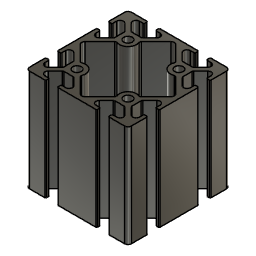
DLLPDF 153030 Cube (Autodesk Fusion 360 design; units mm, degrees)
part number: DLLPDF-153030-350-A
Autodesk Fusion 360 part; units mm, degrees
sketch "Sketch1" plane through (0, 0, 0) normal (0, 0, 1) x (1, 0, 0)
  line L0 (-2.5, 1.5491) -> (-4.7083, 3.7573)
  arc A0 (-4.7083, 3.7573) -> (-6.4, 3.0566) centre (-5.409, 3.0566) ccw
  line L1 (-6.4, 1.95) -> (-6.4, 3.0566)
  arc A1 (-6.65, 1.7) -> (-6.4, 1.95) centre (-6.65, 1.95) ccw
  line L2 (-7.25, 1.7) -> (-6.65, 1.7)
  arc A2 (-7.5, 1.95) -> (-7.25, 1.7) centre (-7.25, 1.95) ccw
  line L3 (-7.5, -6.5) -> (-7.5, -1.95)
  arc A3 (-7.5, -6.5) -> (-6.5, -7.5) centre (-6.5, -6.5) ccw
  line L4 (-6.5, -7.5) -> (-1.95, -7.5)
  arc A4 (-1.95, -7.5) -> (-1.7, -7.25) centre (-1.95, -7.25) ccw
  line L5 (-1.7, -7.25) -> (-1.7, -6.65)
  line L6 (-1.95, -6.4) -> (-3.0566, -6.4)
  arc A5 (-1.7, -6.65) -> (-1.95, -6.4) centre (-1.95, -6.65) ccw
  arc A6 (-3.7573, -4.7083) -> (-3.0566, -6.4) centre (-3.0566, -5.409) ccw
  line L7 (-1.5491, -2.5) -> (-3.7573, -4.7083)
  arc A7 (-6.4, -3.0566) -> (-4.7083, -3.7573) centre (-5.409, -3.0566) ccw
  line L8 (-6.4, -1.95) -> (-6.4, -3.0566)
  line L9 (-7.25, -1.7) -> (-6.65, -1.7)
  arc A8 (-6.4, -1.95) -> (-6.65, -1.7) centre (-6.65, -1.95) ccw
  arc A9 (-7.25, -1.7) -> (-7.5, -1.95) centre (-7.25, -1.95) ccw
  line L10 (-2.5, -1.5491) -> (-4.7083, -3.7573)
  arc A10 (1.6955, -2.6464) -> (1.342, -2.5) centre (1.342, -3) ccw
  arc A11 (-1.342, -2.5) -> (-1.6955, -2.6464) centre (-1.342, -3) ccw
  line L11 (1.342, -2.5) -> (-1.342, -2.5)
  arc A12 (-2.6464, -1.6955) -> (-2.5, -1.342) centre (-3, -1.342) ccw
  arc A13 (-2.5, 1.342) -> (-2.6464, 1.6955) centre (-3, 1.342) ccw
  line L12 (-2.5, -1.342) -> (-2.5, 1.342)
  line L13 (1.5491, -2.5) -> (3.7573, -4.7083)
  arc A14 (1.7, -7.25) -> (1.95, -7.5) centre (1.95, -7.25) ccw
  arc A15 (1.95, -6.4) -> (1.7, -6.65) centre (1.95, -6.65) ccw
  line L14 (1.95, -6.4) -> (3.0566, -6.4)
  arc A16 (3.0566, -6.4) -> (3.7573, -4.7083) centre (3.0566, -5.409) ccw
  line L15 (1.7, -7.25) -> (1.7, -6.65)
  arc A17 (18.0566, -6.4) -> (18.7573, -4.7083) centre (18.0566, -5.409) ccw
  line L16 (16.95, -6.4) -> (18.0566, -6.4)
  arc A18 (16.95, -6.4) -> (16.7, -6.65) centre (16.95, -6.65) ccw
  line L17 (16.7, -7.25) -> (16.7, -6.65)
  arc A19 (16.7, -7.25) -> (16.95, -7.5) centre (16.95, -7.25) ccw
  line L18 (16.5491, -2.5) -> (18.7573, -4.7083)
  arc A20 (19.7083, -3.7573) -> (21.4, -3.0566) centre (20.409, -3.0566) ccw
  line L19 (21.4, -1.95) -> (21.4, -3.0566)
  arc A21 (21.65, -1.7) -> (21.4, -1.95) centre (21.65, -1.95) ccw
  line L20 (22.25, -1.7) -> (21.65, -1.7)
  arc A22 (22.5, -1.95) -> (22.25, -1.7) centre (22.25, -1.95) ccw
  line L21 (22.5, -6.5) -> (22.5, -1.95)
  arc A23 (21.5, -7.5) -> (22.5, -6.5) centre (21.5, -6.5) ccw
  line L22 (21.5, -7.5) -> (16.95, -7.5)
  line L23 (17.5, -1.5491) -> (19.7083, -3.7573)
  arc A24 (17.6464, 1.6955) -> (17.5, 1.342) centre (18, 1.342) ccw
  arc A25 (17.5, -1.342) -> (17.6464, -1.6955) centre (18, -1.342) ccw
  line L24 (17.5, 1.342) -> (17.5, -1.342)
  arc A26 (21.4, 3.0566) -> (19.7083, 3.7573) centre (20.409, 3.0566) ccw
  line L25 (21.4, 1.95) -> (21.4, 3.0566)
  arc A27 (21.4, 1.95) -> (21.65, 1.7) centre (21.65, 1.95) ccw
  line L26 (22.25, 1.7) -> (21.65, 1.7)
  arc A28 (22.25, 1.7) -> (22.5, 1.95) centre (22.25, 1.95) ccw
  line L27 (17.5, 1.5491) -> (19.7083, 3.7573)
  arc A29 (11.2427, -4.7083) -> (11.9434, -6.4) centre (11.9434, -5.409) ccw
  line L28 (13.05, -6.4) -> (11.9434, -6.4)
  arc A30 (13.3, -6.65) -> (13.05, -6.4) centre (13.05, -6.65) ccw
  line L29 (13.3, -7.25) -> (13.3, -6.65)
  arc A31 (13.05, -7.5) -> (13.3, -7.25) centre (13.05, -7.25) ccw
  line L30 (13.4509, -2.5) -> (11.2427, -4.7083)
  arc A32 (16.6955, -2.6464) -> (16.342, -2.5) centre (16.342, -3) ccw
  arc A33 (13.658, -2.5) -> (13.3045, -2.6464) centre (13.658, -3) ccw
  line L31 (16.342, -2.5) -> (13.658, -2.5)
  arc A34 (21.4, 18.0566) -> (19.7083, 18.7573) centre (20.409, 18.0566) ccw
  line L32 (21.4, 16.95) -> (21.4, 18.0566)
  arc A35 (21.4, 16.95) -> (21.65, 16.7) centre (21.65, 16.95) ccw
  line L33 (22.25, 16.7) -> (21.65, 16.7)
  arc A36 (22.25, 16.7) -> (22.5, 16.95) centre (22.25, 16.95) ccw
  line L34 (17.5, 16.5491) -> (19.7083, 18.7573)
  arc A37 (18.7573, 19.7083) -> (18.0566, 21.4) centre (18.0566, 20.409) ccw
  line L35 (16.95, 21.4) -> (18.0566, 21.4)
  arc A38 (16.7, 21.65) -> (16.95, 21.4) centre (16.95, 21.65) ccw
  line L36 (16.7, 22.25) -> (16.7, 21.65)
  arc A39 (16.95, 22.5) -> (16.7, 22.25) centre (16.95, 22.25) ccw
  line L37 (21.5, 22.5) -> (16.95, 22.5)
  arc A40 (22.5, 21.5) -> (21.5, 22.5) centre (21.5, 21.5) ccw
  line L38 (22.5, 21.5) -> (22.5, 16.95)
  line L39 (16.5491, 17.5) -> (18.7573, 19.7083)
  arc A41 (13.3045, 17.6464) -> (13.658, 17.5) centre (13.658, 18) ccw
  arc A42 (16.342, 17.5) -> (16.6955, 17.6464) centre (16.342, 18) ccw
  line L40 (13.658, 17.5) -> (16.342, 17.5)
  arc A43 (11.9434, 21.4) -> (11.2427, 19.7083) centre (11.9434, 20.409) ccw
  line L41 (13.05, 21.4) -> (11.9434, 21.4)
  arc A44 (13.05, 21.4) -> (13.3, 21.65) centre (13.05, 21.65) ccw
  line L42 (13.3, 22.25) -> (13.3, 21.65)
  arc A45 (13.3, 22.25) -> (13.05, 22.5) centre (13.05, 22.25) ccw
  line L43 (13.4509, 17.5) -> (11.2427, 19.7083)
  arc A46 (19.7083, 11.2427) -> (21.4, 11.9434) centre (20.409, 11.9434) ccw
  line L44 (21.4, 13.05) -> (21.4, 11.9434)
  arc A47 (21.65, 13.3) -> (21.4, 13.05) centre (21.65, 13.05) ccw
  line L45 (22.25, 13.3) -> (21.65, 13.3)
  arc A48 (22.5, 13.05) -> (22.25, 13.3) centre (22.25, 13.05) ccw
  line L46 (17.5, 13.4509) -> (19.7083, 11.2427)
  arc A49 (17.6464, 16.6955) -> (17.5, 16.342) centre (18, 16.342) ccw
  arc A50 (17.5, 13.658) -> (17.6464, 13.3045) centre (18, 13.658) ccw
  line L47 (17.5, 16.342) -> (17.5, 13.658)
  arc A51 (-3.0566, 21.4) -> (-3.7573, 19.7083) centre (-3.0566, 20.409) ccw
  line L48 (-1.95, 21.4) -> (-3.0566, 21.4)
  arc A52 (-1.95, 21.4) -> (-1.7, 21.65) centre (-1.95, 21.65) ccw
  line L49 (-1.7, 22.25) -> (-1.7, 21.65)
  arc A53 (-1.7, 22.25) -> (-1.95, 22.5) centre (-1.95, 22.25) ccw
  line L50 (-1.5491, 17.5) -> (-3.7573, 19.7083)
  arc A54 (-4.7083, 18.7573) -> (-6.4, 18.0566) centre (-5.409, 18.0566) ccw
  line L51 (-6.4, 16.95) -> (-6.4, 18.0566)
  arc A55 (-6.65, 16.7) -> (-6.4, 16.95) centre (-6.65, 16.95) ccw
  line L52 (-7.25, 16.7) -> (-6.65, 16.7)
  arc A56 (-7.5, 16.95) -> (-7.25, 16.7) centre (-7.25, 16.95) ccw
  line L53 (-7.5, 21.5) -> (-7.5, 16.95)
  arc A57 (-6.5, 22.5) -> (-7.5, 21.5) centre (-6.5, 21.5) ccw
  line L54 (-6.5, 22.5) -> (-1.95, 22.5)
  line L55 (-2.5, 16.5491) -> (-4.7083, 18.7573)
  arc A58 (-2.6464, 13.3045) -> (-2.5, 13.658) centre (-3, 13.658) ccw
  arc A59 (-2.5, 16.342) -> (-2.6464, 16.6955) centre (-3, 16.342) ccw
  line L56 (-2.5, 13.658) -> (-2.5, 16.342)
  arc A60 (-6.4, 11.9434) -> (-4.7083, 11.2427) centre (-5.409, 11.9434) ccw
  line L57 (-6.4, 13.05) -> (-6.4, 11.9434)
  arc A61 (-6.4, 13.05) -> (-6.65, 13.3) centre (-6.65, 13.05) ccw
  line L58 (-7.25, 13.3) -> (-6.65, 13.3)
  arc A62 (-7.25, 13.3) -> (-7.5, 13.05) centre (-7.25, 13.05) ccw
  line L59 (-2.5, 13.4509) -> (-4.7083, 11.2427)
  arc A63 (3.7573, 19.7083) -> (3.0566, 21.4) centre (3.0566, 20.409) ccw
  line L60 (1.95, 21.4) -> (3.0566, 21.4)
  arc A64 (1.7, 21.65) -> (1.95, 21.4) centre (1.95, 21.65) ccw
  line L61 (1.7, 22.25) -> (1.7, 21.65)
  arc A65 (1.95, 22.5) -> (1.7, 22.25) centre (1.95, 22.25) ccw
  line L62 (1.5491, 17.5) -> (3.7573, 19.7083)
  arc A66 (-1.6955, 17.6464) -> (-1.342, 17.5) centre (-1.342, 18) ccw
  arc A67 (1.342, 17.5) -> (1.6955, 17.6464) centre (1.342, 18) ccw
  line L63 (-1.342, 17.5) -> (1.342, 17.5)
  circle A68 centre (0, 0) radius 1.25
  line L64 (-1.5491, 2.5) -> (-3.7573, 4.7083) construction
  line L65 (-5.842, 6.7929) -> (-1.4771, 2.4281)
  arc A69 (2.318, -0.9363) -> (-0.9363, 2.318) centre (0, 0) ccw
  line L66 (2.4281, -1.4771) -> (6.7929, -5.842)
  arc A70 (2.318, -0.9363) -> (2.4281, -1.4771) centre (2.7816, -1.1236) ccw
  arc A71 (-1.4771, 2.4281) -> (-0.9363, 2.318) centre (-1.1236, 2.7816) ccw
  line L67 (16.4771, 2.4281) -> (20.842, 6.7929)
  arc A72 (15.9363, 2.318) -> (16.4771, 2.4281) centre (16.1236, 2.7816) ccw
  arc A73 (15.9363, 2.318) -> (12.682, -0.9363) centre (15, 0) ccw
  arc A74 (12.5719, -1.4771) -> (12.682, -0.9363) centre (12.2184, -1.1236) ccw
  line L68 (8.2071, -5.842) -> (12.5719, -1.4771)
  line L69 (12.5719, 16.4771) -> (8.2071, 20.842)
  arc A75 (12.682, 15.9363) -> (12.5719, 16.4771) centre (12.2184, 16.1236) ccw
  arc A76 (12.682, 15.9363) -> (15.9363, 12.682) centre (15, 15) ccw
  arc A77 (16.4771, 12.5719) -> (15.9363, 12.682) centre (16.1236, 12.2184) ccw
  line L70 (20.842, 8.2071) -> (16.4771, 12.5719)
  line L71 (-1.4771, 12.5719) -> (-5.842, 8.2071)
  arc A78 (-0.9363, 12.682) -> (-1.4771, 12.5719) centre (-1.1236, 12.2184) ccw
  arc A79 (-0.9363, 12.682) -> (2.318, 15.9363) centre (0, 15) ccw
  arc A80 (2.4281, 16.4771) -> (2.318, 15.9363) centre (2.7816, 16.1236) ccw
  line L72 (6.7929, 20.842) -> (2.4281, 16.4771)
  arc A81 (-5.842, 8.2071) -> (-5.842, 6.7929) centre (-5.1348, 7.5) ccw
  arc A82 (6.7929, -5.842) -> (8.2071, -5.842) centre (7.5, -5.1348) ccw
  arc A83 (20.842, 6.7929) -> (20.842, 8.2071) centre (20.1348, 7.5) ccw
  arc A84 (8.2071, 20.842) -> (6.7929, 20.842) centre (7.5, 20.1348) ccw
  line L73 (-7.5, 13.05) -> (-7.5, 1.95)
  line L74 (1.95, -7.5) -> (13.05, -7.5)
  line L75 (22.5, 1.95) -> (22.5, 13.05)
  line L76 (13.05, 22.5) -> (1.95, 22.5)
  circle A85 centre (15, 0) radius 1.25
  circle A86 centre (0, 15) radius 1.25
  circle A87 centre (15, 15) radius 1.25
  point P0 (7.5, 7.5)
  dimension "d2" = 7.5
  dimension "d3" = 7.5
  dimension "d5" = 360
  dimension "d6" = 2.5
  dimension "d7" = 0.5
  dimension "d9" = 360
  dimension "d10" = 1
  dimension "d12" = 360
  dimension "d15" = 15
  dimension "d16" = 15
  constraint coincident A68.centre A69.centre
  constraint tangent L12 A69
  constraint concentric A68 A69
  constraint collinear L64 L65
  constraint parallel L13 L66
  constraint tangent A69 A70
  constraint tangent L66 A70
  constraint tangent L65 A71
  constraint tangent A69 A71
  constraint equal A70 A71
  constraint collinear L65 L66
  constraint tangent L65 A81
  constraint tangent L71 A81
  constraint tangent L68 A82
  constraint tangent L66 A82
  constraint tangent L67 A83
  constraint tangent L70 A83
  constraint tangent L69 A84
  constraint tangent L72 A84
  constraint coincident A2.start L73.end
  measures "d2" horizontal distance of A68.centre P0
  measures "d3" vertical distance of A68.centre P0
  measures "d6" diameter of A68
  measures "d7" radius of A70
  measures "d10" radius of A81
extrude "Extrude1" add sketch "Sketch1" along normal blind 30
equation "Length = 30 mm"
equation "d3 = d2"
equation "d17 = Length"
